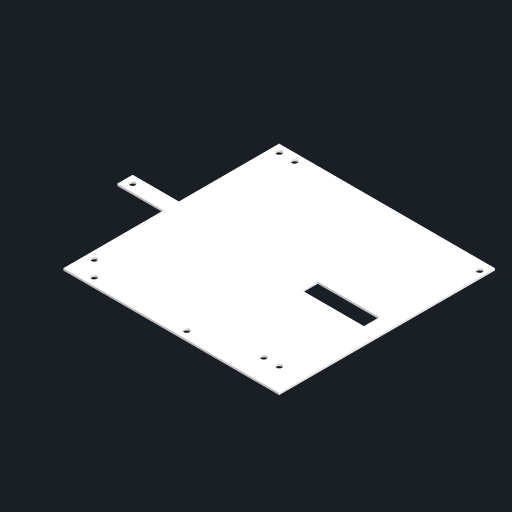
# Autodesk Inventor part: shoot
Saved by Autodesk Inventor 2023 (Build 270158000, 158)
## iProperties
Created: 2023-04-09
Part Number: shoot
Material: ABS Plastic
Document SubType Name: Modeling
Designer: Windows Macbook
Density: 1.06 g/cm^3
Appearance: Smooth - White
Author: Windows Macbook
Autodesk Inventor part; units mm, degrees
ref_plane "YZ Plane" through (0, 0, 0) normal (1, 0, 0) x (0, 1, 0)
ref_plane "XZ Plane" through (0, 0, 0) normal (0, 1, 0) x (-1, 0, 0)
ref_plane "XY Plane" through (0, 0, 0) normal (0, 0, 1) x (1, 0, 0)
sketch "Sketch1" plane through (0, 0, 0) normal (0, 1, 0) x (-1, 0, 0)
  line L0 (0, 0) -> (177.8, 0)
  line L1 (177.8, -177.8) -> (0, -177.8)
  line L2 (0, -177.8) -> (0, 0)
  line L3 (177.8, 0) -> (177.8, -82.55)
  line L4 (177.8, -82.55) -> (215.9, -82.55)
  line L5 (215.9, -82.55) -> (215.9, -95.25)
  line L6 (215.9, -95.25) -> (177.8, -95.25)
  line L7 (177.8, -95.25) -> (177.8, -177.8)
  line L8 (0, 0) -> (0, -88.9)
  line L9 (63.5, -88.9) -> (63.5, -95.25)
  line L10 (12.7, -88.9) -> (12.7, -95.25)
  line L11 (12.7, -95.25) -> (63.5, -95.25)
  line L12 (12.7, -95.25) -> (12.7, -82.55)
  line L13 (12.7, -82.55) -> (63.5, -82.55)
  line L14 (63.5, -82.55) -> (63.5, -95.25)
  dimension "d0" = 177.8
  dimension "d1" = 177.8
  dimension "d39" = 82.55
  dimension "d41" = 12.7
  dimension "d44" = 6.35
  dimension "d45" = 12.7
  constraints: 30 end point, 5 perpendicular, 2 vertical, 1 collinear, 1 horizontal, 1 midpoint, 1 parallel
  measures "d0" distance of L1.start L1.end
  measures "d1" distance of L0.end L1.start
  measures "d39" distance of L0.end L3.end
  measures "d41" distance of L4.end L5.end
  measures "d44" distance of L9.start L9.end
  measures "d45" distance of L8.end L10.start
extrude "Extrusion1" add sketch "Sketch1" along normal blind 1.5875
sketch "Sketch2" plane through (0, 1.5875, 0) normal (0, 1, 0) x (1, 0, 0)
  line L0 (-177.8, 177.8) -> (-177.8, 0) projected
  line L1 (-177.8, 177.8) -> (-177.8, 165.1)
  line L2 (-177.8, 165.1) -> (-165.1, 177.8)
  line L3 (0, 177.8) -> (-177.8, 177.8) projected
  line L4 (-177.8, 177.8) -> (-171.45, 171.45)
  line L5 (-171.45, 171.45) -> (-158.75, 171.45)
  line L6 (-177.8, 0) -> (-165.1, 0)
  line L7 (-177.8, 0) -> (0, 0) projected
  line L8 (0, 177.8) -> (-12.7, 177.8)
  line L9 (0, 0) -> (0, 177.8) projected
  line L10 (0, 0) -> (0, 12.7)
  line L11 (0, 12.7) -> (-12.7, 0)
  line L12 (0, 0) -> (-6.35, 6.35)
  line L13 (-6.35, 6.35) -> (-6.35, 19.05)
  line L14 (-6.35, 19.05) -> (-19.05, 19.05)
  line L15 (-19.05, 19.05) -> (-31.75, 19.05)
  line L16 (-12.7, 177.8) -> (0, 165.1)
  line L17 (0, 177.8) -> (-6.35, 171.45)
  line L18 (-165.1, 0) -> (-177.8, 12.7)
  line L19 (-177.8, 0) -> (-171.45, 6.35)
  line L20 (-171.45, 6.35) -> (-171.45, 19.05)
  line L21 (-171.45, 6.35) -> (-158.75, 6.35)
  line L22 (-6.35, 171.45) -> (-6.35, 169.799)
  line L23 (-6.35, 169.799) -> (-4.699, 169.799)
  line L24 (-215.9, 82.55) -> (-177.8, 82.55) projected
  line L25 (-215.9, 82.55) -> (-203.2, 95.25)
  line L26 (-177.8, 95.25) -> (-215.9, 95.25) projected
  line L27 (-215.9, 82.55) -> (-197.9395, 82.55) construction
  line L28 (-203.2, 95.25) -> (-215.9, 95.25)
  line L29 (-215.9, 95.25) -> (-203.2, 82.55)
  point P0 (-209.55, 88.9)
  dimension "d4" = 12.7
  dimension "d5" = 45
  dimension "d6" = 12.7
  dimension "d7" = 12.7
  dimension "d12" = 12.7
  dimension "d28" = 1.651
  dimension "d42" = 45
  constraints: 48 end point, 11 point on line, 7 coincident, 5 midpoint, 4 horizontal, 4 perpendicular, 3 vertical, 1 collinear, 1 equal length
  measures "d4" distance of L0.start L1.end
  measures "d5" angle of L2 L1
  measures "d6" distance of L4.end L5.end
  measures "d7" distance of L0.end L6.end
  measures "d12" distance of L7.end L10.end
  measures "d28" distance of L17.end L22.end
  measures "d42" angle of L27 L25
hole "Hole2" at (-171.45, 1.5875, -171.45) at (-158.75, 1.5875, -171.45) at (-19.05, 1.5875, -19.05) at (-31.75, 1.5875, -19.05) at (-171.45, 1.5875, -19.05) at (-158.75, 1.5875, -6.35) at (-4.699, 1.5875, -169.799) at (-209.55, 1.5875, -88.9) direction (0, -1, 0) diameter 4.7625 end through all
sketch "Sketch3" plane through (0, 1.5875, 0) normal (0, 1, 0) x (1, 0, 0)
  line L0 (0, 0) -> (0, 12.7)
  line L1 (0, 0) -> (0, 177.8) projected
  line L2 (0, 12.7) -> (-12.7, 0)
  line L3 (-177.8, 0) -> (0, 0) projected
  line L4 (-12.7, 0) -> (0, 0)
  line L5 (0, 0) -> (-6.35, 6.35)
  line L6 (-6.35, 6.35) -> (-82.55, 6.35)
  dimension "d29" = 12.7
  dimension "d30" = 45
  dimension "d31" = 76.2
  constraints: 10 end point, 2 point on line, 1 coincident, 1 collinear, 1 midpoint, 1 parallel
  measures "d29" distance of L0.start L0.end
  measures "d30" angle of L2 L0
  measures "d31" distance of L5.end L6.end
hole "Hole3" at (-82.55, 1.5875, -6.35) direction (0, -1, 0) diameter 4.7625 end through all
body "Solid1"
